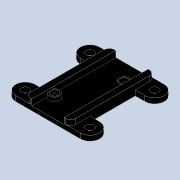
# Autodesk Inventor part: DCDC Converter Mount
Saved by Autodesk Inventor 2022 (Build 260153000, 153)
## iProperties
Created: 2022-02-05
Part Number: DCDC Converter Mount
Material: Generic
Document SubType Name: Modeling
Designer: Coy
Density: 1 g/cm^3
Appearance: Anodized - Black
Author: Coy
Autodesk Inventor part; units mm, degrees
ref_plane "YZ Plane" through (0, 0, 0) normal (1, 0, 0) x (0, 1, 0)
sketch "Sketch1" plane through (0, 0, 0) normal (0, 1, 0) x (-1, 0, 0)
  line L0 (0, 0) -> (24, 0)
  line L1 (24, 0) -> (24, -54)
  line L2 (24, -54) -> (0, -54)
  line L3 (0, -54) -> (0, 0)
  circle A0 centre (21.5, -9) radius 1.5
  circle A1 centre (2.5, -44) radius 1.5
  line L4 (24.5, -54.5) -> (24.5, 0.5)
  line L5 (24.5, 0.5) -> (-0.5, 0.5)
  line L6 (-0.5, 0.5) -> (-0.5, -54.5)
  line L7 (-0.5, -54.5) -> (24.5, -54.5)
  line L8 (29.5, 5.5) -> (29.5, -59.5)
  line L9 (29.5, -59.5) -> (-5.5, -59.5)
  line L10 (-5.5, -59.5) -> (-5.5, 5.5)
  line L11 (-5.5, 5.5) -> (29.5, 5.5)
  dimension "d0" = 24
  dimension "d1" = 54
  dimension "d2" = 3
  dimension "d3" = 3
  dimension "d4" = 9
  dimension "d5" = 2.5
  dimension "d6" = 2.5
  dimension "d7" = 10
  dimension "d8" = 0.5
  dimension "d9" = 5
  constraints: 24 end point, 6 parallel, 3 perpendicular, 2 centre point, 1 horizontal, 6 other
  measures "d0" distance of L1.end L2.end
  measures "d1" distance of L0.end L1.end
  measures "d2" diameter of A0
  measures "d3" diameter of A1
  measures "d4" distance from line of L0 A0.centre
  measures "d5" distance from line of L1 A0.centre
  measures "d6" distance from line of L3 A1.centre
  measures "d7" distance from line of L2 A1.centre
  measures "d8" distance between parallel lines of L1 L4
  measures "d9" distance between parallel lines of L4 L8
extrude "Extrusion1" add sketch "Sketch1" against normal blind 1.7 contours L8 L9 L10 L11
ref_plane "Work Plane1" through (0, -1.7, 0) normal (0, 1, 0) x (1, 0, 0)
sketch "Sketch2" plane through (0, -1.7, 0) normal (0, 1, 0) x (1, 0, 0)
  line L0 (0, 0) -> (-24, 0)
  line L1 (-24, 0) -> (-24, 54)
  line L2 (-24, 54) -> (0, 54)
  line L3 (0, 54) -> (0, 0)
  circle A0 centre (-21.5, 9) radius 1.5
  circle A1 centre (-2.5, 44) radius 1.5
  line L4 (-24.5, 54.5) -> (-24.5, -0.5)
  line L5 (-24.5, -0.5) -> (0.5, -0.5)
  line L6 (0.5, -0.5) -> (0.5, 54.5)
  line L7 (0.5, 54.5) -> (-24.5, 54.5)
  line L8 (-29.5, -5.5) -> (-29.5, 59.5)
  line L9 (-29.5, 59.5) -> (5.5, 59.5)
  line L10 (5.5, 59.5) -> (5.5, -5.5)
  line L11 (5.5, -5.5) -> (-29.5, -5.5)
  circle A2 centre (-21.5, 9) radius 4
  circle A3 centre (-2.5, 44) radius 4
  point P0 (-24.5, 6.3542)
  point P1 (-24.5, 11.6458)
  point P2 (0.5, 46.6458)
  point P3 (0.5, 41.3542)
  dimension "d13" = 24
  dimension "d14" = 54
  dimension "d15" = 3
  dimension "d16" = 3
  dimension "d17" = 9
  dimension "d18" = 2.5
  dimension "d19" = 2.5
  dimension "d20" = 10
  dimension "d21" = 0.5
  dimension "d22" = 5
  dimension "d23" = 8
  dimension "d24" = 8
  constraints: 24 end point, 6 parallel, 4 centre point, 3 perpendicular, 2 coincident, 6 other
  measures "d13" distance of L1.end L2.end
  measures "d14" distance of L0.end L1.end
  measures "d15" diameter of A0
  measures "d16" diameter of A1
  measures "d17" distance from line of L0 A0.centre
  measures "d18" distance from line of L1 A0.centre
  measures "d19" distance from line of L3 A1.centre
  measures "d20" distance from line of L2 A1.centre
  measures "d21" distance between parallel lines of L1 L4
  measures "d22" distance between parallel lines of L4 L8
  measures "d23" diameter of A2
  measures "d24" diameter of A3
extrude "Extrusion2" add sketch "Sketch2" against normal blind 3 contours A3 L3 | L3 A3 L6 | A2 L4 L1 | L1 A2 | L6 A3 | A2 L4 | L8 L9 L10 L11
sketch "Sketch3" plane through (0, -4.7, 0) normal (0, -1, 0) x (1, 0, 0)
  line L0 (5.5, -59.5) -> (5.5, 5.5) projected
  line L1 (5.5, 5.5) -> (-29.5, 5.5) projected
  line L2 (-29.5, 5.5) -> (-29.5, -59.5) projected
  line L3 (-29.5, -59.5) -> (5.5, -59.5) projected
  point P0 (0, 0)
extrude "Extrusion3" add sketch "Sketch3" along normal blind 3.3
ref_plane "Work Plane2" through (0, -8, 0) normal (0, 1, 0) x (1, 0, 0)
sketch "Sketch4" plane through (0, -8, 0) normal (0, 1, 0) x (1, 0, 0)
  line L0 (-37, 2) -> (13, 2) construction
  line L1 (13, 2) -> (13, 52) construction
  line L2 (13, 52) -> (-37, 52) construction
  line L3 (-37, 52) -> (-37, 2) construction
  line L4 (0.5, -0.5) -> (-24.5, -0.5) construction
  line L5 (-12, -0.5) -> (-12, 54.5) construction
  line L6 (-24.5, 54.5) -> (0.5, 54.5) construction
  line L7 (-29.5, 59.5) -> (-29.5, -5.5) projected
  line L8 (-29.5, 27) -> (5.5, 27) construction
  line L9 (5.5, -5.5) -> (5.5, 59.5) projected
  circle A0 centre (-37, 2) radius 3
  circle A1 centre (-37, 52) radius 3
  circle A2 centre (13, 52) radius 3
  circle A3 centre (13, 2) radius 3
  circle A4 centre (-37, 2) radius 7.5
  line L10 (-29.5, -5.5) -> (5.5, -5.5) projected
  circle A5 centre (-37, 52) radius 7.5
  circle A6 centre (13, 52) radius 7.5
  circle A7 centre (13, 2) radius 7.5
  line L11 (5.5, 59.5) -> (-29.5, 59.5) projected
  line L12 (5.5, -5.5) -> (13, -5.5)
  line L13 (5.5, 59.5) -> (13, 59.5)
  line L14 (13, 44.5) -> (5.5, 44.5)
  line L15 (13, 9.5) -> (5.5, 9.5)
  line L16 (-29.5, -5.5) -> (-37, -5.5)
  line L17 (-37, 9.5) -> (-29.5, 9.5)
  line L18 (-37, 44.5) -> (-29.5, 44.5)
  line L19 (-37, 59.5) -> (-29.5, 59.5)
  point P0 (0, 0)
  dimension "d30" = 50
  dimension "d31" = 50
  dimension "d32" = 25
  dimension "d33" = 25
  dimension "d34" = 6
  dimension "d35" = 6
  dimension "d36" = 6
  dimension "d37" = 6
  constraints: 28 end point, 12 point on line, 8 centre point, 8 point on circle, 8 tangent, 7 coincident, 4 midpoint, 4 parallel, 3 perpendicular, 1 horizontal
  measures "d30" distance of L2.end L1.end
  measures "d31" distance of L1.end L0.end
  measures "d32" distance between parallel lines of L5 L3
  measures "d33" distance between parallel lines of L8 L0
  measures "d34" diameter of A0
  measures "d35" diameter of A1
  measures "d36" diameter of A2
  measures "d37" diameter of A3
extrude "Extrusion4" add sketch "Sketch4" along normal blind 4 contours L7 A5 L19 | A5 | L7 L18 A5 | L13 A6 L9 | A6 L14 L9 | A6 | L7 A4 L17 | A4 | L7 L16 A4 | L15 A7 L9 | A7 L12 L9 | A7
fillet "Fillet1" radius 4 6 edges at (5.5, -2.85, -59.5) (5.5, -0.85, -59.5) (-29.5, -2, -59.5) (-29.5, -2, 5.5) (5.5, -0.85, 5.5) (5.5, -2.85, 5.5)
chamfer "Chamfer1" distance 1.5 angle 45 2 edges at (-4, -1.7, -44) (-23, -1.7, -9)
sketch "Sketch5" plane through (-2.5, -4.7, -44) normal (0, 1, 0) x (1, 0, 0)
  circle A0 centre (-19, -35) radius 1.5 projected
  circle A1 centre (0, 0) radius 1.5 projected
  point P0 (2.5, -44)
extrude "Extrusion5" cut sketch "Sketch5" against normal through all
sketch "Sketch6" plane through (0, 0, 0) normal (0, 1, 0) x (1, 0, 0)
  line L0 (-24.5, 54.5) -> (0.5, 54.5) projected
  line L1 (0.5, 54.5) -> (0.5, 59.563)
  line L2 (1.5, 59.5) -> (-25.5, 59.5) projected
  line L3 (-24.5, 54.5) -> (-24.5, 59.5)
  line L4 (0.5, -0.5) -> (-24.5, -0.5) projected
  line L5 (0.5, -0.5) -> (0.5, -5.5)
  line L6 (-25.5, -5.5) -> (1.5, -5.5) projected
  line L7 (-24.5, -0.5) -> (-24.5, -5.5)
  point P0 (0, 0)
  point P1 (0.5, 59.5)
  constraints: 8 end point, 4 point on line, 2 perpendicular, 1 parallel
extrude "Extrusion6" cut sketch "Sketch6" against normal up to surface (4.7 mm away)
equation "\"d3\" = d2"
equation "\"d6\" = d5"
equation "\"d16\" = d15"
equation "\"d19\" = d18"
equation "\"d24\" = d23"
equation "\"d32\" = 0.5 * d30"
equation "\"d33\" = 0.5 * d31"
equation "\"d35\" = d34"
equation "\"d36\" = d34"
equation "\"d37\" = d34"
body "Solid1"
